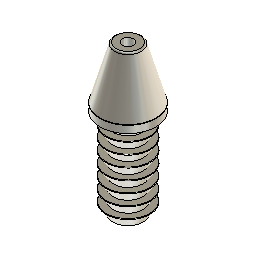
hoseNozzle (Autodesk Fusion 360 design; units mm, degrees)
part number: 2025-10-06-19-48-03-451
Autodesk Fusion 360 part; units mm, degrees
sketch "Sketch4" plane through (0, 0, 0) normal (0, 1, 0) x (1, 0, 0)
  line L0 (0, 0) -> (0, 40) construction
  line L1 (-4, 40) -> (-6, 40) construction
  line L2 (-6, 40) -> (-6, 37) construction
  line L3 (-6, 37) -> (-6, 34) construction
  line L4 (-4.1187, 39.8219) -> (-5.8964, 37.1555)
  line L5 (-5.8131, 37) -> (-4, 37)
  line L6 (-4, 37) -> (-5.8964, 34.1555)
  line L7 (-5.8131, 34) -> (-4, 34)
  line L8 (-3.7859, 40) -> (-2.5, 40)
  line L9 (-2.5, 40) -> (-2.5, 15)
  line L10 (-6, 34) -> (-6, 31) construction
  line L11 (-6, 31) -> (-6, 28) construction
  line L12 (-4, 34) -> (-5.8964, 31.1555)
  line L13 (-4, 31) -> (-5.8131, 31)
  line L14 (-4, 31) -> (-5.8964, 28.1555)
  line L15 (-6, 28) -> (-6, 25) construction
  line L16 (-6, 25) -> (-6, 22) construction
  line L17 (-5.8131, 28) -> (-4, 28)
  line L18 (-4, 28) -> (-5.8964, 25.1555)
  line L19 (-5.8131, 25) -> (-4, 25)
  line L20 (-4, 25) -> (-5.8964, 22.1555)
  arc A0 (-5.8964, 25.1555) -> (-5.8131, 25) centre (-5.8131, 25.1) ccw
  arc A1 (-5.8964, 28.1555) -> (-5.8131, 28) centre (-5.8131, 28.1) ccw
  arc A2 (-5.8964, 31.1555) -> (-5.8131, 31) centre (-5.8131, 31.1) ccw
  arc A3 (-5.8964, 34.1555) -> (-5.8131, 34) centre (-5.8131, 34.1) ccw
  arc A4 (-5.8964, 37.1555) -> (-5.8131, 37) centre (-5.8131, 37.1) ccw
  arc A5 (-3.7859, 40) -> (-4.1187, 39.8219) centre (-3.7859, 39.6) ccw
  line L21 (-6, 22) -> (-6, 19) construction
  line L22 (-6, 19) -> (-6, 16) construction
  line L23 (-5.8131, 22) -> (-4, 22)
  line L24 (-4, 22) -> (-5.8964, 19.1555)
  line L25 (-5.8131, 19) -> (-4, 19)
  line L26 (-4, 19) -> (-6, 16)
  arc A6 (-5.8964, 22.1555) -> (-5.8131, 22) centre (-5.8131, 22.1) ccw
  arc A7 (-5.8964, 19.1555) -> (-5.8131, 19) centre (-5.8131, 19.1) ccw
  line L27 (-6, 16) -> (-7.5, 16)
  line L28 (-7.5, 16) -> (-7.5, 14.07)
  line L29 (0, 0) -> (-1.5, 0) construction
  line L30 (-2.5, 15) -> (-1.5, 0)
  line L31 (-1.5, 0) -> (-3.1228, 0)
  line L32 (-3.6036, 0.3626) -> (-7.4808, 13.9327)
  arc A8 (-3.6036, 0.3626) -> (-3.1228, 0) centre (-3.1228, 0.5) ccw
  arc A9 (-7.5, 14.07) -> (-7.4808, 13.9327) centre (-7, 14.07) ccw
  point P0 (-7.5, 14)
  point P1 (-3.5, 0)
  dimension "d10" = 40
  dimension "d11" = 4
  dimension "d12" = 3
  dimension "d13" = 3
  dimension "d14" = 2
  dimension "d15" = 1.5
  dimension "d16" = 25
  dimension "d17" = 3
  dimension "d18" = 3
  dimension "d19" = 3
  dimension "d20" = 3
  dimension "d21" = 2
  dimension "d22" = 2
  dimension "d23" = 0.1
  dimension "d24" = 0.4
  dimension "d25" = 3
  dimension "d26" = 3
  dimension "d27" = 2
  dimension "d28" = 2
  dimension "d29" = 0.1
  dimension "d30" = 0.1
  dimension "d31" = 1.5
  dimension "d32" = 2
  dimension "d33" = 1.5
  dimension "d34" = 2
  dimension "d35" = 0.5
  constraint coincident L0.start L29.start
  constraint vertical L0
  constraint perpendicular L0 L1
  constraint perpendicular L1 L2
  constraint parallel L2 L3
  constraint perpendicular L3 L5
  constraint perpendicular L3 L7
  constraint parallel L1 L8
  constraint perpendicular L8 L9
  constraint perpendicular L7 L10
  constraint parallel L10 L11
  constraint perpendicular L10 L13
  constraint parallel L12 L14
  constraint parallel L11 L15
  constraint parallel L15 L16
  constraint perpendicular L11 L17
  constraint perpendicular L15 L19
  constraint coincident L15.end L18
  constraint coincident L15.end L19
  constraint tangent L18 A0
  constraint tangent L19 A0
  constraint coincident L11.end L14
  constraint coincident L11.end L17
  constraint tangent L14 A1
  constraint tangent L17 A1
  constraint equal A0 A1
  constraint coincident L10.end L12
  constraint coincident L10.end L13
  constraint tangent L12 A2
  constraint tangent L13 A2
  constraint equal A0 A2
  constraint coincident L3.end L7
  constraint coincident L3.end L6
  constraint tangent L7 A3
  constraint tangent L6 A3
  constraint equal A0 A3
  constraint coincident L2.end L4
  constraint coincident L2.end L5
  constraint tangent L4 A4
  constraint tangent L5 A4
  constraint equal A0 A4
  constraint coincident L1.start L8
  constraint coincident L1.start L4
  constraint tangent L8 A5
  constraint tangent L4 A5
  constraint parallel L16 L21
  constraint parallel L21 L22
  constraint perpendicular L16 L23
  constraint perpendicular L21 L25
  constraint coincident L16.end L20
  constraint coincident L16.end L23
  constraint tangent L20 A6
  constraint tangent L23 A6
  constraint coincident L21.end L24
  constraint coincident L21.end L25
  constraint tangent L24 A7
  constraint tangent L25 A7
  constraint perpendicular L22 L27
  constraint perpendicular L27 L28
  constraint perpendicular L0 L29
  constraint perpendicular L0 L31
  constraint coincident P1 L31
  constraint coincident P1 L32
  constraint tangent L31 A8
  constraint tangent L32 A8
  constraint coincident P0 L28
  constraint coincident P0 L32
  constraint tangent L28 A9
  constraint tangent L32 A9
  constraint equal A8 A9
  measures "d10" distance of L0.start L0.end
  measures "d11" distance of L0.end L1.start
  measures "d12" distance of L1.end L2.end
  measures "d13" distance of L2.end L3.end
  measures "d14" distance of L2.end L5.end
  measures "d15" distance of L1.start L8.end
  measures "d16" distance of L8.end L9.end
  measures "d17" distance of L3.end L10.end
  measures "d18" distance of L10.end L11.end
  measures "d19" distance of L11.end L15.end
  measures "d20" distance of L15.end L16.end
  measures "d21" distance of L11.end L17.end
  measures "d22" distance of L15.end L19.end
  measures "d23" radius of A0
  measures "d24" radius of A5
  measures "d25" distance of L16.end L21.end
  measures "d26" distance of L21.end L22.end
  measures "d27" distance of L16.end L23.end
  measures "d28" distance of L21.end L25.end
  measures "d29" radius of A6
  measures "d30" radius of A7
  measures "d31" distance of L22.end L27.end
  measures "d32" distance of L27.end P0
  measures "d33" distance of L0.start L29.end
  measures "d34" distance of L29.end P1
  measures "d35" radius of A8
revolve "Revolve1" add sketch "Sketch4" angle 360 about axis through (0, 0, 0) along (0, 0, -1)
move_body "Move1" bodies 1 to x (1, 0, 0) y (0, 1, 0) z (0, 0, 1) at (0, 0, 40)
